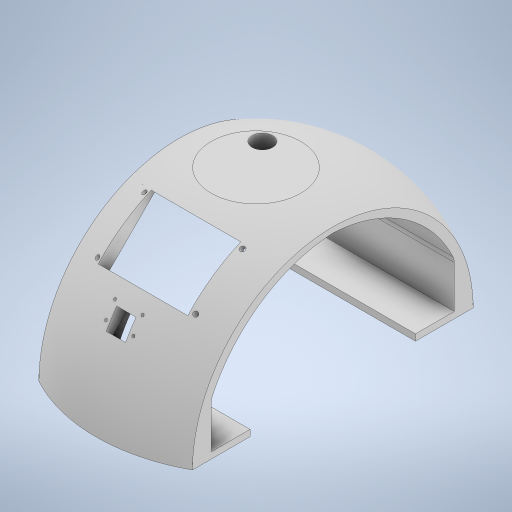
# Autodesk Inventor part: newhead
Saved by Autodesk Inventor 2023 (Build 270158000, 158)
## iProperties
Created: 2022-11-23
Part Number: newhead
Material: 一般
Document SubType Name: Modeling
Designer: yuta
Density: 1 g/cm^3
Appearance: 既定
Author: yuta
Autodesk Inventor part; units mm, degrees
ref_plane "YZ Plane" through (0, 0, 0) normal (1, 0, 0) x (0, 1, 0)
ref_plane "XZ Plane" through (0, 0, 0) normal (0, 1, 0) x (-1, 0, 0)
ref_plane "XY Plane" through (0, 0, 0) normal (0, 0, 1) x (1, 0, 0)
sketch "スケッチ1" plane through (0, 0, 0) normal (0, 0, 1) x (1, 0, 0)
  line L0 (0, 0) -> (-125, 0)
  line L1 (0, 0) -> (125, 0) construction
  arc A0 (-35, 120) -> (-125, 0) centre (0, 0) ccw
  line L2 (-125, 0) -> (0, 125) construction
  line L3 (-125, 0) -> (51.7767, 0) construction
  line L4 (0, 125) -> (0, 0)
  line L5 (0, 120) -> (-35, 120)
  line L6 (0, 120) -> (35, 120) construction
  dimension "d0" = 125
  dimension "d1" = 180
  dimension "d2" = 45
  dimension "d3" = 125
  dimension "d4" = 120
  dimension "d5" = 180
  constraints: 14 end point, 4 horizontal, 3 equal length, 2 point on circle, 1 centre point, 1 point on line, 1 vertical
  measures "d0" distance of L0.start L0.end
  measures "d1" angle of L0 L1
  measures "d2" angle of L3 L2
  measures "d3" radius of A0
  measures "d4" distance of L0.start L5.start
  measures "d5" angle of L5 L6
revolve "回転1" add sketch "スケッチ1" angle 360 about axis through (0, 125, 0) along (0, -1, 0)
sketch "スケッチ2" plane through (0, 0, 0) normal (0, -1, 0) x (1, 0, 0)
  line L0 (60, -125) -> (-60, -125)
  line L1 (-60, -125) -> (-60, 125)
  line L2 (-60, 125) -> (60, 125)
  line L3 (60, 125) -> (60, -125)
  line L4 (60, -125) -> (-60, 125) construction
  line L5 (-60, -125) -> (60, 125) construction
  circle A0 centre (0, 0) radius 125
  point P0 (60, 109.6586)
  point P1 (60, -109.6586)
  point P2 (-60, 109.6586)
  point P3 (-60, -109.6586)
  dimension "d7" = 120
  dimension "d8" = 250
  constraints: 12 end point, 2 midpoint, 2 parallel, 1 centre point, 1 coincident, 1 horizontal, 1 perpendicular
  measures "d7" distance of L1.end L2.end
  measures "d8" distance of L0.end L1.end
extrude "押し出し1" cut sketch "スケッチ2" against normal blind 200 contours L3 A0 | A0 L1
sketch "スケッチ3" plane through (-60, 0, -109.6586) normal (-1, 0, 0) x (0, 0, 1)
  line L0 (219.3171, 0) -> (0, 0) projected
  line L1 (219.3171, 0) -> (109.6586, 109.6586)
  arc A0 (219.3171, 0) -> (0, 0) centre (109.6586, 0) ccw projected
  line L2 (219.3171, 0) -> (374.3977, 0) construction
  line L3 (109.6586, 109.6586) -> (0, 0)
  dimension "d11" = 135
  constraints: 6 end point, 1 equal length, 1 horizontal, 1 perpendicular, 1 point on circle
  measures "d11" angle of L2 L1
extrude "押し出し2" cut sketch "スケッチ3" against normal blind 200 contours L0 L3 L1
sketch "スケッチ4" plane through (60, 0, 109.6586) normal (0, -0.7071068, -0.7071068) x (-1, 0, 0)
  line L0 (95, 72.5403) -> (25, 72.5403)
  line L1 (25, 72.5403) -> (25, 122.5403)
  line L2 (25, 122.5403) -> (95, 122.5403)
  line L3 (95, 122.5403) -> (95, 72.5403)
  line L4 (95, 72.5403) -> (25, 122.5403) construction
  line L5 (25, 72.5403) -> (95, 122.5403) construction
  line L6 (0, 0) -> (0, 155.0806) projected
  ellipse E0 centre (60, 77.5403) end of major axis (-65, 77.5403) minor radius 88.3883 (0, 0) -> (120, 0) ccw projected
  point P0 (60, 77.5403)
  point P1 (60, 97.5403)
  dimension "d14" = 70
  dimension "d15" = 50
  dimension "d16" = 60
  dimension "d17" = 20
  constraints: 12 end point, 2 midpoint, 2 parallel, 1 horizontal, 1 perpendicular, 1 other
  measures "d14" distance of L1.end L2.end
  measures "d15" distance of L0.end L1.end
  measures "d16" distance from line of L6 point (60, 97.54)
  measures "d17" distance of point (60, 77.54) point (60, 97.54)
extrude "押し出し3" cut sketch "スケッチ4" against normal blind 200
sketch "スケッチ5" plane through (60, 0, 109.6586) normal (0, -0.7071068, -0.7071068) x (-1, 0, 0)
  line L0 (67.5, 42.5403) -> (52.5, 42.5403)
  line L1 (52.5, 42.5403) -> (52.5, 57.5403)
  line L2 (52.5, 57.5403) -> (67.5, 57.5403)
  line L3 (67.5, 57.5403) -> (67.5, 42.5403)
  line L4 (67.5, 42.5403) -> (52.5, 57.5403) construction
  line L5 (52.5, 42.5403) -> (67.5, 57.5403) construction
  line L6 (25, 72.5403) -> (25, 122.5403) projected
  line L7 (95, 72.5403) -> (25, 72.5403) projected
  point P0 (60, 77.5403)
  point P1 (60, 50.0403)
  dimension "d20" = 15
  dimension "d21" = 15
  dimension "d22" = 42.5
  dimension "d23" = 15
  constraints: 12 end point, 2 midpoint, 2 parallel, 1 horizontal, 1 perpendicular
  measures "d20" distance of L1.end L2.end
  measures "d21" distance of L0.end L1.end
  measures "d22" distance between parallel lines of L6 L3
  measures "d23" distance between parallel lines of L7 L2
extrude "押し出し4" cut sketch "スケッチ5" against normal blind 200
sketch "スケッチ6" plane through (60, 0, 109.6586) normal (0, -0.7071068, -0.7071068) x (-1, 0, 0)
  line L0 (72.75, 37.7903) -> (47.25, 37.7903)
  line L1 (47.25, 37.7903) -> (47.25, 62.2903)
  line L2 (47.25, 62.2903) -> (72.75, 62.2903)
  line L3 (72.75, 62.2903) -> (72.75, 37.7903)
  line L4 (72.75, 37.7903) -> (47.25, 62.2903) construction
  line L5 (47.25, 37.7903) -> (72.75, 62.2903) construction
  line L6 (52.5, 42.5403) -> (52.5, 57.5403) projected
  line L7 (67.5, 42.5403) -> (52.5, 42.5403) projected
  point P0 (60, 77.5403)
  point P1 (60, 50.0403)
  dimension "d26" = 25.5
  dimension "d27" = 24.5
  dimension "d28" = 5.25
  dimension "d29" = 4.75
  constraints: 12 end point, 2 midpoint, 2 parallel, 1 horizontal, 1 perpendicular
  measures "d26" distance of L1.end L2.end
  measures "d27" distance of L0.end L1.end
  measures "d28" distance between parallel lines of L6 L1
  measures "d29" distance between parallel lines of L7 L0
extrude "押し出し5" cut sketch "スケッチ6" against normal blind 35
sketch "スケッチ7" plane through (60, 24.7487, 134.4073) normal (0, -0.7071068, -0.7071068) x (-1, 0, 0)
  line L0 (47.25, 62.2903) -> (72.75, 62.2903) projected
  line L1 (47.25, 37.7903) -> (47.25, 62.2903) projected
  line L2 (72.75, 62.2903) -> (72.75, 37.7903) projected
  point P0 (60, 77.5403)
  point P1 (49.25, 60.2903)
  point P2 (70.75, 60.2903)
  point P3 (49.25, 47.7903)
  point P4 (47.25, 50.0403)
  point P5 (70.75, 47.7903)
  dimension "d32" = 2
  dimension "d33" = 2
  dimension "d34" = 2
  dimension "d35" = 2
  dimension "d36" = 12.5
  dimension "d37" = 2
  dimension "d48" = 12.5
  dimension "d49" = 2
  constraints: 1 midpoint
  measures "d32" distance from line of L0 point (49.25, 60.29)
  measures "d33" distance from line of L1 point (49.25, 60.29)
  measures "d34" distance from line of L2 point (70.75, 60.29)
  measures "d35" distance from line of L0 point (70.75, 60.29)
  measures "d36" distance of point (49.25, 47.79) point (49.25, 60.29)
  measures "d37" horizontal distance of point (47.25, 50.04) point (49.25, 47.79)
  measures "d48" distance of point (70.75, 60.29) point (70.75, 47.79)
  measures "d49" distance from line of L2 point (70.75, 47.79)
hole "穴1" at (10.75, 67.3804, 91.7756) at (-10.75, 67.3804, 91.7756) at (10.75, 58.5416, 100.6144) at (-10.75, 58.5416, 100.6144) direction (0, 0.7071068, 0.7071068) diameter 2 depth 12 tip angle 118
sketch "スケッチ8" plane through (60, 0, 109.6586) normal (0, -0.7071068, -0.7071068) x (-1, 0, 0)
  line L0 (72.75, 37.7903) -> (47.25, 37.7903) projected
  line L1 (47.25, 37.7903) -> (72.75, 37.7903)
  line L2 (72.75, 37.7903) -> (72.75, 17.7903)
  line L3 (72.75, 17.7903) -> (47.25, 17.7903)
  line L4 (47.25, 17.7903) -> (47.25, 37.7903)
  point P0 (60, 77.5403)
  dimension "d45" = 20
  constraints: 8 end point, 2 parallel, 1 horizontal, 1 perpendicular
  measures "d45" distance of L1.end L2.end
extrude "押し出し6" cut sketch "スケッチ8" against normal blind 25
sketch "スケッチ9" plane through (0, 0, 0) normal (0, -1, 0) x (1, 0, 0)
  arc A0 (60, 109.6586) -> (-60, 109.6586) centre (0, 0) ccw projected
  line L0 (60, 109.6586) -> (-60, 109.6586)
  line L1 (-60, 109.6586) -> (-60, 89.6586)
  line L2 (-60, 89.6586) -> (60, 89.6586)
  line L3 (60, 89.6586) -> (60, 109.6586)
  line L4 (0, 0) -> (9.1314, 0)
  line L5 (-60, 0) -> (60, 0) projected
  line L6 (60, -109.6586) -> (-60, -109.6586)
  line L7 (-60, -109.6586) -> (-60, -89.6586)
  line L8 (-60, -89.6586) -> (60, -89.6586)
  line L9 (60, -89.6586) -> (60, -109.6586)
  point P0 (0, 0)
  dimension "d50" = 120
  dimension "d51" = 20
  constraints: 18 end point, 4 symmetric about line, 2 parallel, 1 horizontal, 1 perpendicular, 1 point on line
  measures "d50" distance of L2.end L1.end
  measures "d51" distance of L1.end L0.end
extrude "押し出し7" add sketch "スケッチ9" against normal blind 5 contours L3 L2 L1 L0 | L6 L7 L8 L9
fillet "フィレット1" radius 7 2 edges at (0, 5, -104.6586) (0, 5, 104.6586)
fillet "フィレット2" radius 10 1 edges at (0, 109.6586, 0)
sketch "スケッチ11" plane through (12.75, 44.0459, 65.6127) normal (0, -0.7071068, -0.7071068) x (-1, 0, 0)
  line L0 (57.6, 10) -> (-28.9, 10)
  line L1 (-28.9, 10) -> (-28.9, 60.5)
  line L2 (-28.9, 60.5) -> (57.6, 60.5)
  line L3 (57.6, 60.5) -> (57.6, 10)
  line L4 (57.6, 10) -> (-28.9, 60.5) construction
  line L5 (-28.9, 10) -> (57.6, 60.5) construction
  line L6 (47.75, 10.25) -> (-22.25, 10.25) projected
  line L7 (-22.25, 10.25) -> (-22.25, 60.25) projected
  point P0 (12.75, 15.25)
  point P1 (14.35, 35.25)
  dimension "d56" = 86.5
  dimension "d57" = 50.5
  dimension "d58" = 25
  dimension "d62" = 6.65
  constraints: 12 end point, 2 midpoint, 2 parallel, 1 horizontal, 1 perpendicular
  measures "d56" distance of L1.end L2.end
  measures "d57" distance of L0.end L1.end
  measures "d58" distance from line of L6 point (14.35, 35.25)
  measures "d62" distance between parallel lines of L1 L7
extrude "押し出し8" cut sketch "スケッチ11" against normal blind 30
sketch "スケッチ12" plane through (12.75, 65.2591, 86.8259) normal (0, -0.7071068, -0.7071068) x (-1, 0, 0)
  line L0 (-28.9, 60.5) -> (57.6, 60.5) projected
  line L1 (-28.9, 10) -> (-28.9, 60.5) projected
  line L2 (57.6, 10) -> (-28.9, 10) projected
  line L3 (47.75, 10.25) -> (47.75, 60.25) projected
  point P0 (12.75, 15.25)
  point P1 (-25.7, 57.3)
  point P2 (-25.7, 13.2)
  point P3 (50.95, 57.3)
  point P4 (50.95, 13.2)
  dimension "d63" = 3.2
  dimension "d64" = 3.2
  dimension "d65" = 3.2
  dimension "d66" = 3.2
  dimension "d67" = 3.2
  dimension "d75" = 3.2
  measures "d63" distance from line of L0 point (-25.7, 57.3)
  measures "d64" distance from line of L1 point (-25.7, 57.3)
  measures "d65" distance from line of L2 point (-25.7, 13.2)
  measures "d66" distance from line of L1 point (-25.7, 13.2)
  measures "d67" distance from line of point (50.95, 57.3) L3
  measures "d75" distance from line of point (50.95, 57.3) L0
hole "穴2" at (38.45, 105.7763, 46.3086) at (38.45, 74.5929, 77.4921) at (-38.2, 105.7763, 46.3086) at (-38.2, 74.5929, 77.4921) direction (0, 0.7071068, 0.7071068) diameter 3.4 depth 12 tip angle 118
sketch "スケッチ13" plane through (60, 0, 109.6586) normal (1, 0, 0) x (0, 0, -1)
  line L0 (20, 0) -> (0, 0) projected
  line L1 (20, 0) -> (45, 0)
  line L2 (45, 0) -> (45, 5)
  line L3 (45, 5) -> (20, 5)
  line L4 (20, 5) -> (20, 0)
  line L5 (109.6586, 0) -> (109.6586, 17.5385)
  line L6 (199.3171, 0) -> (174.3171, 0)
  line L7 (174.3171, 0) -> (174.3171, 5)
  line L8 (174.3171, 5) -> (199.3171, 5)
  line L9 (199.3171, 5) -> (199.3171, 0)
  dimension "d76" = 25
  dimension "d77" = 5
  constraints: 18 end point, 4 symmetric about line, 2 parallel, 1 horizontal, 1 perpendicular, 1 vertical
  measures "d76" distance of L3.end L2.end
  measures "d77" distance of L2.end L1.end
extrude "押し出し9" add sketch "スケッチ13" against normal blind 120
sketch "スケッチ14" plane through (0, 120, 0) normal (0, 1, 0) x (1, 0, 0)
  circle A0 centre (-15, 20) radius 8
  point P0 (0, 0)
  dimension "d80" = 16
  dimension "d81" = 20
  dimension "d82" = 15
  constraints: 1 centre point
  measures "d80" diameter of A0
  measures "d81" vertical distance of point (0, 0) A0.centre
  measures "d82" horizontal distance of point (0, 0) A0.centre
extrude "押し出し10" cut sketch "スケッチ14" against normal blind 120
sketch "スケッチ15" plane through (60, 0, 0) normal (1, 0, 0) x (0, 0, -1)
  line L0 (64.6586, 0) -> (64.6586, 5) projected
  arc A0 (89.6586, 5) -> (92.9164, 16.7422) centre (87.9666, 11.7924) ccw projected
  line L1 (64.6586, 5) -> (94.9666, 5)
  line L2 (94.9666, 5) -> (94.9666, 11.7924)
  line L3 (94.9666, 11.7924) -> (64.6586, 11.7924)
  line L4 (64.6586, 11.7924) -> (64.6586, 5)
  arc A1 (-92.9164, 16.7422) -> (-94.8075, 10.3082) centre (-87.9666, 11.7924) ccw projected
  line L5 (64.6586, 5) -> (-94.9666, 5)
  line L6 (-94.9666, 5) -> (-94.9666, 11.7924)
  line L7 (-94.9666, 11.7924) -> (64.6586, 11.7924)
  line L8 (64.6586, 11.7924) -> (64.6586, 5)
  line L9 (-94.9666, 11.7924) -> (94.9666, 11.7924)
  line L10 (94.9666, 11.7924) -> (94.9666, 40.3933)
  line L11 (94.9666, 40.3933) -> (-94.9666, 40.3933)
  line L12 (-94.9666, 40.3933) -> (-94.9666, 11.7924)
  arc A2 (7.0711, 102.5875) -> (-7.0711, 102.5875) centre (0, 95.5164) ccw projected
  arc A3 (0, 105.5164) -> (-94.9666, 40.3933) centre (5.7922, -4.7348) ccw
  line L13 (0, 11.7924) -> (0, 21.8917)
  arc A4 (94.9666, 40.3933) -> (0, 105.5164) centre (-5.7922, -4.7348) ccw
  point P0 (0, 0)
  point P1 (89.6586, 5)
  point P2 (94.9666, 11.7924)
  constraints: 26 end point, 7 point on circle, 6 parallel, 3 horizontal, 3 perpendicular, 2 centre point, 1 midpoint, 1 point on line, 1 symmetric about line, 1 vertical, 1 other
extrude "押し出し11" cut sketch "スケッチ15" against normal blind 120 contours L1 L4 L3 A0 | A0 L2 L1 | L3 L7 L12 L11 L10 | L5 L6 L7 L4 | L11 A3 A4
fillet "フィレット3" radius 10 3 edges at (0, 40.3933, -94.9666) (36.375, 40.3933, 94.9666) (-36.375, 40.3933, 94.9666)
